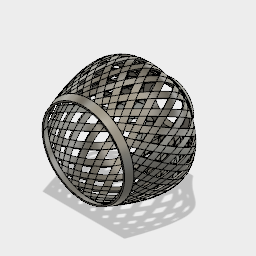
amphold (v1~recovered) (Autodesk Fusion 360 design; units mm, degrees)
Autodesk Fusion 360 part; units mm, degrees
sketch "Sketch1" plane through (0, 0, 0) normal (0, 1, 0) x (1, 0, 0)
  line L0 (0, 0) -> (0, 130)
  line L1 (0, 0) -> (-60, 0)
  line L2 (0, 130) -> (-30.4967, 130)
  spline S0 degree 5 poles (-60, 0) (-61.8229, 4.9602) (-65.2312, 14.5951) (-69.6315, 28.1911) (-74.0504, 44.5774) (-77.0123, 62.0128) (-77.2254, 76.2748) (-74.557, 87.4094) (-69.0295, 95.7889) (-61.035, 102.4291) (-51.3775, 109.0259) (-43.0224, 115.7156) (-36.7311, 122.205) (-32.5694, 127.2773) (-30.4967, 130) knots 0 0 0 0 0 0 0.1 0.2 0.3 0.4 0.5 0.6 0.7 0.8 0.9 1 1 1 1 1 1
  line L3 (-42.7888, 113.8529) -> (-18.2046, 146.1471)
  point P0 (-70.6268, 92.565)
  dimension "d1" = 130
  dimension "d2" = 60
  dimension "d3" = 30.4967
  measures "d1" distance of L0.start L0.end
  measures "d2" distance of L0.start L1.end
  measures "d3" distance of L0.end L2.end
revolve "Revolve1" add sketch "Sketch1" angle 360 about axis through (0, 0, 0) along (0, 0, -1) makes body 1
split "Split1" by plane through (0, 0, -122) normal (0, 0, -1) bodies 1 makes body 2 at (5.4209, 13.3151, -130)
sketch "Sketch2" plane through (0, 0, -130) normal (0, 0, -1) x (-1, 0, 0)
  circle A0 centre (0, 0) radius 30.4967
  circle A1 centre (0, 0) radius 25.9155
extrude "Extrude1" cut sketch "Sketch2" against normal blind 10 contours A1 bodies 2
shell "Shell1" thickness 2 removed faces 2 at (-28.282, -12.1475, 0) at (2.1901, -14.2845, -122) on bodies 1
split "Split2" by plane through (0, 0, -10) normal (0, 0, 1) bodies 1 makes body 3 at (53.0385, -30.5992, -3.3875)
sketch "Sketch3" plane through (0, 0, 0) normal (1, 0, 0) x (0, 0, -1)
  line L0 (10, 63.5619) -> (10, -63.5619)
  line L1 (122, -37.1974) -> (122, 37.1974)
  line L2 (122, 23.5698) -> (10, -31.7304)
  line L3 (122, 14.7098) -> (10, -40.5904)
  line L4 (10, 0) -> (122, 0)
  line L5 (10, 0) -> (122, 0)
extrude "Extrude2" cut sketch "Sketch3" along normal mid plane 270 contours L0 L2 L3 L4 L5 | L1 L2 L3 L4 L5 keep common part bodies 1 makes body 4 at (57.2438, -30.1697, -19.7927)
pattern_circular "C-Pattern1" count 22 over 360 about axis through (0, 0, 1.75) along (0, 0, 1) of bodies 4 makes body 5 at (63.4101, -12.8396, -19.7597) makes body 6 at (43.4399, 37.8309, -102.1986) makes body 7 at (60.2874, 23.5048, -19.7923) makes body 8 at (51.2276, 39.5175, -19.7645) makes body 9 at (38.0126, 52.3613, -19.7831) makes body 10 at (21.7207, 60.9499, -19.7835) makes body 11 at (3.6742, 64.5978, -19.776) makes body 12 at (-43.6223, 37.6001, -102.2086) makes body 13 at (-31.8341, 56.3295, -19.7771) makes body 14 at (-44.08, -1.6252, -112.5905) makes body 15 at (-57.2438, 30.1697, -19.7927) makes body 16 at (-63.4101, 12.8396, -19.7597) makes body 17 at (-43.4399, -37.8309, -102.1986) makes body 18 at (-60.2874, -23.5048, -19.7923) makes body 19 at (-51.2276, -39.5175, -19.7645) makes body 20 at (-38.0126, -52.3613, -19.7831) makes body 21 at (-21.7207, -60.9499, -19.7835) makes body 22 at (-3.6742, -64.5978, -19.776) makes body 23 at (43.6223, -37.6001, -102.2086) makes body 24 at (31.8341, -56.3295, -19.7771) makes body 25 at (44.08, 1.6252, -112.5905)
pattern_circular "C-Pattern2" count 22 over 360 about axis through (0, 0, 1.75) along (0, 0, 1) of bodies 1 makes body 26 at (-46.8729, -44.938, -20.5057) makes body 27 at (-32.3156, -56.3231, -20.508) makes body 28 at (-15.1422, -63.1466, -20.5126) makes body 29 at (3.269, -64.8511, -20.5024) makes body 30 at (21.411, -61.2998, -20.4963) makes body 31 at (37.8123, -52.7872, -20.5) makes body 32 at (51.1507, -40.0025, -20.5083) makes body 33 at (60.3488, -23.9741, -20.5117) makes body 34 at (64.6574, -5.9971, -20.5071) makes body 35 at (63.7252, 12.4659, -20.5012) makes body 36 at (57.6264, 29.9189, -20.4925) makes body 37 at (46.8729, 44.938, -20.5057) makes body 38 at (32.3156, 56.3231, -20.508) makes body 39 at (15.1422, 63.1466, -20.5126) makes body 40 at (-3.269, 64.8511, -20.5024) makes body 41 at (-21.411, 61.2998, -20.4963) makes body 42 at (-37.8123, 52.7872, -20.5) makes body 43 at (-51.1507, 40.0025, -20.5083) makes body 44 at (-60.3488, 23.9741, -20.5117) makes body 45 at (-64.6574, 5.9971, -20.5071) makes body 46 at (-63.7252, -12.4659, -20.5012)
